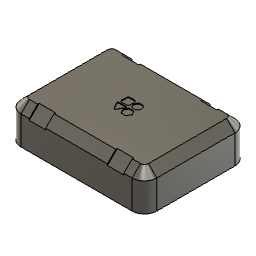
Bento Revised - Flat (Autodesk Fusion 360 design; units mm, degrees)
Autodesk Fusion 360 part; units mm, degrees
note: some values were not read from the file. Chosen so that the rebuilt part matches the saved one: which face or edge a step refers to.
sketch "Sketch1" plane through (0, 0, 0) normal (0, 1, 0) x (1, 0, 0)
  line L0 (82.5, 62.5) -> (-82.5, 62.5)
  line L1 (-82.5, 62.5) -> (-82.5, -62.5)
  line L2 (-82.5, -62.5) -> (82.5, -62.5)
  line L3 (82.5, -62.5) -> (82.5, 62.5)
  line L4 (82.5, 62.5) -> (-82.5, -62.5) construction
  line L5 (-82.5, 62.5) -> (82.5, -62.5) construction
  dimension "d1" = 165
  dimension "d2" = 125
  constraint horizontal L0
  constraint perpendicular L0 L1
  constraint parallel L0 L2
  constraint parallel L1 L3
  constraint coincident L4 origin
  constraint coincident L5 origin
  measures "d1" distance of L0.start L0.end
  measures "d2" distance of L0.start L2.end
extrude "Extrude1" add sketch "Sketch1" along normal blind 88 makes body 1
sketch "Sketch2" plane through (0, 0, 62.5) normal (0, 0, 1) x (1, 0, 0)
  line L0 (-82.5, 0) -> (82.5, 0)
  line L1 (82.5, 0) -> (82.5, 88)
  line L2 (82.5, 88) -> (-82.5, 88)
  line L3 (-82.5, 88) -> (-82.5, 0)
  line L4 (-28.95, 71.8572) -> (-48.25, 83)
  line L5 (-48.25, 83) -> (-67.55, 71.8572)
  line L6 (-67.55, 71.8572) -> (-67.55, 49.5714)
  line L7 (-67.55, 49.5714) -> (-48.25, 38.4286)
  line L8 (-48.25, 38.4286) -> (-28.95, 49.5714)
  line L9 (-28.95, 49.5714) -> (-28.95, 71.8572)
  circle A0 centre (-48.25, 60.7143) radius 22.2857 construction
  line L10 (-48.25, 60.7143) -> (-38.6, 44) construction
  line L11 (-48.25, 16.1428) -> (-28.95, 5)
  line L12 (-28.95, 5) -> (-9.65, 16.1428)
  line L13 (-9.65, 16.1428) -> (-9.65, 38.4286)
  line L14 (-9.65, 38.4286) -> (-28.95, 49.5714)
  line L15 (-28.95, 49.5714) -> (-48.25, 38.4286)
  line L16 (-48.25, 38.4286) -> (-48.25, 16.1428)
  line L17 (-28.95, 49.5714) -> (-9.65, 38.4286)
  line L18 (-9.65, 38.4286) -> (9.65, 49.5714)
  line L19 (9.65, 49.5714) -> (9.65, 71.8572)
  line L20 (9.65, 71.8572) -> (-9.65, 83)
  line L21 (-9.65, 83) -> (-28.95, 71.8572)
  line L22 (-28.95, 71.8572) -> (-28.95, 49.5714)
  line L23 (-9.65, 16.1428) -> (9.65, 5)
  line L24 (9.65, 5) -> (28.95, 16.1428)
  line L25 (28.95, 16.1428) -> (28.95, 38.4286)
  line L26 (28.95, 38.4286) -> (9.65, 49.5714)
  line L27 (9.65, 49.5714) -> (-9.65, 38.4286)
  line L28 (-9.65, 38.4286) -> (-9.65, 16.1428)
  line L29 (9.65, 49.5714) -> (28.95, 38.4286)
  line L30 (28.95, 38.4286) -> (48.25, 49.5714)
  line L31 (48.25, 49.5714) -> (48.25, 71.8572)
  line L32 (48.25, 71.8572) -> (28.95, 83)
  line L33 (28.95, 83) -> (9.65, 71.8572)
  line L34 (9.65, 71.8572) -> (9.65, 49.5714)
  line L35 (28.95, 16.1428) -> (48.25, 5)
  line L36 (48.25, 5) -> (67.55, 16.1428)
  line L37 (67.55, 16.1428) -> (67.55, 38.4286)
  line L38 (67.55, 38.4286) -> (48.25, 49.5714)
  line L39 (48.25, 49.5714) -> (28.95, 38.4286)
  line L40 (28.95, 38.4286) -> (28.95, 16.1428)
  line L41 (0, 77.4286) -> (0, 10.5714) construction
  line L42 (0, 0) -> (0, 88) construction
  line L43 (-82.5, 44) -> (82.5, 44) construction
  line L44 (-82.5, 44) -> (82.5, 44)
  line L45 (67.55, 38.4286) -> (67.55, 44)
  line L46 (57.9, 44) -> (57.9, 10.5714)
  point P0 (-48.25, 60.7143)
  dimension "d5" = 38.6
  dimension "d8" = 38.6
  dimension "d9" = 38.6
  dimension "d10" = 14.95
  dimension "d12" = 5
  dimension "d13" = 78
  constraint coincident P0 A0.centre
  constraint coincident L4.start A0
  constraint vertical L6
  constraint midpoint L8 L10.end
  constraint midpoint L20 L41.start
  constraint midpoint L23 L41.end
  constraint coincident L42.start origin
  constraint midpoint L2 L42.end
  constraint collinear L41 L42
  constraint midpoint L3 L43.start
  constraint midpoint L1 L43.end
  constraint midpoint L41 L43
  constraint coincident L43 L45.end
  constraint perpendicular L43 L45
  constraint midpoint L38 L46.start
  constraint coincident L36 L46.end
  constraint vertical L46
  measures "d5" distance of L6 L9
  measures "d10" distance of L1 L37
  measures "d12" distance of L2 L20.end
  measures "d13" vertical distance of L20.end L23.end
extrude "Extrude2" add sketch "Sketch2" against normal blind 105 from surface at -10 separate body contours L7 L8 L15 L44 | L4 L5 L6 L7 L8 L9 L15 L22 L44 | L8 L11 L12 L13 L14 L15 L16 L17 L28 L44 | L8 L14 L15 L17 L44 | L30 L38 L39 L44 | L25 L30 L35 L36 L39 L40 L44 L46 | L36 L37 L38 L46 | L9 L14 L17 L18 L19 L20 L21 L22 L27 L34 L44 | L14 L17 L18 L27 L44 | L19 L26 L29 L30 L31 L32 L33 L34 L39 L44 | L26 L29 L30 L39 L44 | L13 L18 L23 L24 L25 L26 L27 L28 L29 L40 L44 | L18 L26 L27 L29 L44 makes body 2
fillet "Fillet1" radius 5 18 edges at (28.95, 83, 0) (48.25, 71.8572, 0) (48.25, 49.5714, 0) (67.55, 38.4286, 0) (67.55, 16.1428, 0) (48.25, 5, 0) (-9.65, 83, 0) (9.65, 71.8572, 0) (-28.95, 71.8572, 0) (-48.25, 83, 0) (-67.55, 71.8572, 0) (-67.55, 49.5714, 0) (-48.25, 38.4286, 0) (-48.25, 16.1428, 0) (-28.95, 5, 0) (-9.65, 16.1428, 0) (9.65, 5, 0) (28.95, 16.1428, 0) on bodies 2
fillet "Fillet5" radius 15 4 edges at (82.5, 44, 62.5) (-82.5, 44, 62.5) (82.5, 44, -62.5) (-82.5, 44, -62.5) on bodies 1
chamfer "Chamfer4" distance 10.16 angle 45 16 edges at (78.1066, 88, 58.1066) (82.5, 88, 0) (78.1066, 88, -58.1066) (0, 88, -62.5) (-78.1066, 88, -58.1066) (-82.5, 88, 0) (-78.1066, 88, 58.1066) (0, 88, 62.5) (82.5, 0, 0) (78.1066, 0, -58.1066) (0, 0, -62.5) (-78.1066, 0, -58.1066) (-82.5, 0, 0) (-78.1066, 0, 58.1066) (0, 0, 62.5) (78.1066, 0, 58.1066) on bodies 1
combine "Combine1" operation cut target body 1 tool bodies 2
extrude "Extrude3" cut sketch "Sketch2" against normal blind 105 from surface at -10 contours L38 L44 L45 | L36 L37 L38 L46 bodies 1
extrude "Extrude4" cut sketch "Sketch2" against normal blind 125 contours L1 L2 L3 L4 L5 L6 L7 L20 L21 L31 L32 L33 L38 L44 | L4 L5 L6 L7 L8 L9 L15 L22 L44 | L8 L14 L15 L17 L44 | L30 L38 L39 L44 | L9 L14 L17 L18 L19 L20 L21 L22 L27 L34 L44 | L19 L26 L29 L30 L31 L32 L33 L34 L39 L44 | L18 L26 L27 L29 L44 bodies 1
fillet "Fillet3" radius 5 1 edges at (67.55, 16.1428, 0) on bodies 1
sketch "Sketch4" plane through (-82.5, 0, 0) normal (-1, 0, 0) x (0, 0, 1)
  line L0 (47.5, 44) -> (-47.5, 44)
  line L1 (0, 0) -> (-52.5, 0)
  line L2 (-62.5, 10) -> (-62.5, 44)
  line L3 (-62.5, 44) -> (62.5, 44)
  line L4 (62.5, 44) -> (62.5, 10)
  line L5 (52.5, 0) -> (0, 0)
  line L6 (54.3333, 42.5) -> (54.3333, 3.8333)
  line L7 (-54.8333, 42.5) -> (54.3333, 42.5)
  line L8 (-54.8333, 4.3333) -> (-54.8333, 42.5)
  line L9 (0, 0.0714) -> (-50.5714, 0.0714)
  line L10 (50.5714, 0.0714) -> (0, 0.0714)
  line L11 (54.3333, 42.5) -> (54.3333, 44)
  line L12 (-54.8333, 42.5) -> (-54.8333, 44)
  line L13 (-47.5, 44) -> (-47.5, 10.16)
  line L14 (-47.5, 10.16) -> (47.5, 10.16)
  line L15 (47.5, 10.16) -> (47.5, 44)
  line L16 (54.3333, 3.8333) -> (50.5714, 0.0714)
  line L17 (62.5, 10) -> (52.5, 0)
  line L18 (-54.8333, 4.3333) -> (-50.5714, 0.0714)
  line L19 (-62.5, 10) -> (-52.5, 0)
  line L20 (54.3333, 3.8333) -> (62.5, 12)
  line L21 (50.5714, 0.0714) -> (50.5, 0)
  line L22 (-50.5714, 0.0714) -> (-50.5, 0)
  line L23 (-54.8333, 4.3333) -> (-62.5, 12)
  point P0 (-62.5, 0)
  point P1 (62.5, 0)
  point P2 (0, 44)
  dimension "d38" = 44
  dimension "d39" = 44
  dimension "d40" = 125
  dimension "d70" = 10
  dimension "d71" = 2
  dimension "d72" = 45
  dimension "d73" = 45
  dimension "d74" = 10
  dimension "d75" = 2
  constraint coincident L1.start L5.end
  constraint horizontal L1
  constraint perpendicular L1 L2
  constraint perpendicular L2 L3
  constraint perpendicular L0 L4
  constraint perpendicular L4 L5
  constraint coincident P0 L2
  constraint coincident P0 L1
  constraint coincident P1 L5
  constraint coincident P1 L4
  constraint coincident L3 L11.end
  constraint perpendicular L3 L11
  constraint midpoint L3 P2
  constraint coincident L3 L12.end
  constraint perpendicular L3 L12
  constraint parallel L4 L6
  constraint parallel L3 L7
  constraint parallel L2 L8
  constraint parallel L1 L9
  constraint parallel L5 L10
  constraint coincident L4 L20.end
  constraint parallel L16 L20
  constraint coincident L5 L21.end
  constraint parallel L16 L21
  constraint coincident L1 L22.end
  constraint perpendicular L21 L22
  constraint coincident L2 L23.end
  constraint parallel L18 L23
  constraint parallel L17 L20
  constraint parallel L19 L23
  measures "d38" distance of L3.end P1
  measures "d39" distance of P0 L2.end
  measures "d40" distance of L2 L4
  measures "d70" vertical distance of L2.start L1.end
  measures "d71" distance of L2.start L23.end
  measures "d72" angle of L1 L19
  measures "d73" angle of L5 L17
  measures "d74" vertical distance of L5.start L4.end
  measures "d75" distance of L4.end L20.end
extrude "Extrude7" cut sketch "Sketch4" against normal blind 20 from surface at -25 contours L4 L5 L16 L17 L20 L21 | L1 L2 L18 L19 L22 L23 bodies 1
extrude "Extrude8" cut sketch "Sketch4" against normal blind 20 from surface at -120 contours L4 L5 L16 L17 L20 L21 | L1 L2 L18 L19 L22 L23 bodies 1
sketch "Sketch5" plane through (0, 44, 0) normal (0, 1, 0) x (-1, 0, 0)
  line L0 (-67.55, -52.5) -> (-67.55, 52.5)
  line L1 (-67.55, 52.5) -> (57.9, 52.5)
  line L2 (67.5, 62.5) -> (-67.5, 62.5)
  arc A0 (-67.5, 62.5) -> (-82.5, 47.5) centre (-67.5, 47.5) ccw
  line L3 (-82.5, 47.5) -> (-82.5, -47.5)
  arc A1 (-82.5, -47.5) -> (-67.5, -62.5) centre (-67.5, -47.5) ccw
  line L4 (-67.55, -25) -> (-82.5, -25)
  line L5 (-82.5, -25) -> (-82.5, 25)
  line L6 (-82.5, 25) -> (-67.55, 25)
  line L7 (-67.55, 25) -> (-67.55, -25)
  line L8 (0, -52.5) -> (0, 52.5)
  line L9 (82.5, 25) -> (67.55, 25)
  line L10 (67.55, 25) -> (67.55, -25)
  line L11 (67.55, -25) -> (82.5, -25)
  line L12 (82.5, -25) -> (82.5, 25)
  arc A2 (67.5, -62.5) -> (82.5, -47.5) centre (67.5, -47.5) ccw
  line L13 (82.5, -47.5) -> (82.5, 47.5)
  arc A3 (82.5, 47.5) -> (67.5, 62.5) centre (67.5, 47.5) ccw
  line L14 (57.9, 52.5) -> (57.9, -52.5)
  line L15 (0, -62.5) -> (0, -45)
  line L16 (0, 52.5) -> (0, 62.5)
  line L17 (67.55, 25) -> (67.55, 52.5)
  line L18 (67.55, 52.5) -> (0, 52.5)
  line L19 (0, -45) -> (-67.55, -45)
  line L20 (-67.55, -45) -> (-67.55, -25)
  line L21 (67.55, -25) -> (67.55, -45)
  line L22 (67.55, -45) -> (0, -45)
  line L23 (-67.55, 0) -> (-82.5, 0)
  line L24 (67.55, 0) -> (82.5, 0)
  line L25 (-67.5, -62.5) -> (67.5, -62.5)
  line L26 (57.9, -52.5) -> (-67.55, -52.5)
  line L27 (67.5, 62.5) -> (0, 62.5)
  dimension "d52" = 50
  constraint horizontal L4
  constraint vertical L5
  constraint horizontal L6
  constraint vertical L7
  constraint coincident L3 L5.end
  constraint coincident L0 L4.start
  constraint symmetric L4.start L8 L10.end
  constraint symmetric L4.end L8 L11.end
  constraint symmetric L5.end L8 L9.start
  constraint symmetric L6.end L8 L9.end
  constraint coincident L8 L15.end
  constraint coincident L1 L8.end
  constraint coincident L8 L16.start
  constraint midpoint L2 L16.end
  constraint perpendicular L1 L17
  constraint perpendicular L16 L18
  constraint perpendicular L0 L19
  constraint perpendicular L4 L20
  constraint midpoint L5 L23.end
  constraint midpoint L13 L24.end
  constraint coincident L10 L24.start
  constraint perpendicular L10 L24
  constraint coincident L0 L23.start
  constraint midpoint L3 L23.end
  constraint midpoint L7 L23.start
  constraint midpoint L15.start L25
  constraint horizontal L22
  constraint coincident L2.start A3.end
  measures "d52" distance of L4 L6
extrude "Extrude9" [suppressed]
extrude "Extrude11" [suppressed]
sketch "Sketch7" plane through (-67.55, 0, 0) normal (1, 0, 0) x (0, 0, -1)
  line L0 (-52.5, 44) -> (0, 44)
  line L1 (0, 44) -> (0, 49)
  line L2 (0, 49) -> (-52.5, 49)
  line L3 (-52.5, 49) -> (-52.5, 44)
  line L4 (-52.5, 49) -> (52.5, 49)
  line L5 (52.5, 49) -> (52.5, 39)
  line L6 (52.5, 39) -> (-52.5, 39)
  line L7 (-52.5, 39) -> (-52.5, 49)
  dimension "d82" = 105
  constraint horizontal L4
  constraint vertical L5
  constraint horizontal L6
  constraint vertical L7
  constraint coincident L2.end L3.start
  measures "d82" distance of L2.end L4.end
extrude "Extrude12" [suppressed]
chamfer "Chamfer1" [suppressed]
chamfer "Chamfer7" [suppressed]
chamfer "Chamfer8" [suppressed]
copy_body "CopyPasteBodies1" bodies 1 makes body 3
sketch "Sketch1 (2)" plane through (0, 0, 0) normal (0, 1, 0) x (1, 0, 0) in component "Logo v7 (1)"
  line L0 (5.725, 5.925) -> (-5.725, 5.925) construction
  line L1 (-5.725, 5.925) -> (-5.725, -5.925) construction
  line L2 (-5.725, -5.925) -> (5.725, -5.925) construction
  line L3 (5.725, -5.925) -> (5.725, 5.925) construction
  line L4 (5.725, 5.925) -> (-5.725, -5.925) construction
  line L5 (-5.725, 5.925) -> (5.725, -5.925) construction
  line L6 (-10.725, 10.925) -> (-0.725, 10.925)
  line L7 (-0.725, 10.925) -> (-0.725, 0.925)
  line L8 (-0.725, 0.925) -> (-10.725, 0.925)
  line L9 (-10.725, 0.925) -> (-10.725, 10.925)
  line L10 (-10.725, 10.925) -> (-0.725, 0.925) construction
  line L11 (-0.725, 10.925) -> (-10.725, 0.925) construction
  circle A0 centre (5.725, 5.925) radius 5
  circle A1 centre (-8.725, 8.925) radius 2
  circle A2 centre (-2.725, 8.925) radius 2
  circle A3 centre (-8.725, 2.925) radius 2
  circle A4 centre (-2.725, 2.925) radius 2
  line L12 (2.4132, -0.925) -> (-0.4735, -5.925)
  line L13 (-0.4735, -5.925) -> (2.4132, -10.925)
  line L14 (2.4132, -10.925) -> (8.1868, -10.925)
  line L15 (8.1868, -10.925) -> (11.0735, -5.925)
  line L16 (11.0735, -5.925) -> (8.1868, -0.925)
  line L17 (8.1868, -0.925) -> (2.4132, -0.925)
  line L18 (-5.725, -11.925) -> (0.6259, -0.925)
  line L19 (0.6259, -0.925) -> (-12.0759, -0.925)
  line L20 (-12.0759, -0.925) -> (-5.725, -11.925)
  circle A5 centre (-5.725, -4.5917) radius 7.3333 construction
  circle A6 centre (5.3, -5.925) radius 5.7735 construction
  circle A7 centre (-10.3438, -1.925) radius 1
  circle A8 centre (-1.1062, -1.925) radius 1
  circle A9 centre (-5.725, -9.925) radius 1
  circle A10 centre (0.5657, -5.925) radius 0.9
  circle A11 centre (2.9329, -1.825) radius 0.9
  circle A12 centre (7.6671, -1.825) radius 0.9
  circle A13 centre (10.0343, -5.925) radius 0.9
  circle A14 centre (7.6671, -10.025) radius 0.9
  circle A15 centre (2.9329, -10.025) radius 0.9
  line L21 (0.6259, -0.925) -> (2.4132, -0.925) construction
  point P0 (-5.725, 5.925)
  point P1 (5.3, -5.925)
  point P2 (-5.725, -4.5917)
  dimension "d1_2" = 11.45
  dimension "d2_2" = 11.85
  dimension "d3_2" = 10
  dimension "d4_2" = 10
  dimension "d5_2" = 10
  dimension "d10_2" = 4
  dimension "d11_1" = 4
  dimension "d12_2" = 4
  dimension "d13_2" = 4
  dimension "d14_2" = 0.425
  dimension "d15_2" = 10
  dimension "d18_1" = 1.8
  dimension "d19_2" = 1.8
  dimension "d20_2" = 1.8
  dimension "d21_2" = 1.8
  dimension "d22_2" = 1.8
  dimension "d23_2" = 1.8
  dimension "d24_2" = 2
  dimension "d25_2" = 2
  dimension "d26_1" = 2
  dimension "d29_2" = 9
  constraint perpendicular L0 L1
  constraint parallel L0 L2
  constraint parallel L1 L3
  constraint horizontal L0
  constraint coincident L4 origin
  constraint coincident L5 origin
  constraint perpendicular L6 L7
  constraint parallel L6 L8
  constraint parallel L7 L9
  constraint horizontal L6
  constraint coincident L10 P0
  constraint coincident L11 P0
  constraint coincident P0 L0.end
  constraint coincident L0.start L3.end
  constraint tangent L9 A1
  constraint tangent L6 A1
  constraint tangent L6 A2
  constraint tangent L7 A2
  constraint tangent L9 A3
  constraint tangent L8 A3
  constraint tangent L8 A4
  constraint tangent L7 A4
  constraint coincident P2 A5.centre
  constraint coincident L19.end A5
  constraint coincident P1 A6.centre
  constraint coincident L16.end A6
  constraint coincident L2 P1
  constraint horizontal L17
  constraint horizontal L19
  constraint coincident L1 P2
  constraint tangent L20 A7
  constraint tangent L19 A7
  constraint tangent L19 A8
  constraint tangent L18 A8
  constraint tangent L18 A9
  constraint tangent L20 A9
  constraint tangent L13 A10
  constraint tangent L12 A10
  constraint tangent L12 A11
  constraint tangent L17 A11
  constraint tangent L17 A12
  constraint tangent L16 A12
  constraint tangent L16 A13
  constraint tangent L15 A13
  constraint tangent L15 A14
  constraint tangent L14 A14
  constraint tangent L14 A15
  constraint tangent L13 A15
  constraint parallel L17 L21
  measures "d1_2" distance of L1 L3
  measures "d2_2" vertical distance of L0.start L2.end
  measures "d3_2" vertical distance of L6.start L8.end
  measures "d4_2" horizontal distance of L6.start L6.end
  measures "d5_2" diameter of A0
  measures "d10_2" diameter of A1
  measures "d11_1" diameter of A2
  measures "d12_2" diameter of A3
  measures "d13_2" diameter of A4
  measures "d14_2" horizontal distance of L2.end P1
  measures "d15_2" distance of L14 L17
  measures "d18_1" diameter of A10
  measures "d19_2" diameter of A11
  measures "d20_2" diameter of A12
  measures "d21_2" diameter of A13
  measures "d22_2" diameter of A14
  measures "d23_2" diameter of A15
  measures "d24_2" diameter of A8
  measures "d25_2" diameter of A7
  measures "d26_1" diameter of A9
  measures "d29_2" distance of L19 A9.centre
extrude "Extrude1'" add sketch "Sketch1 (2)" along normal blind 1 separate body contours L6 L7 L8 L9 A1 A2 A3 A4 | A1 | A2 | A3 | A4 | A0 | L12 L13 L14 L15 L16 L17 A10 A11 A12 A13 A14 A15 | A11 | A10 | A12 | A15 | A13 | A14 | L18 L19 L20 A7 A8 A9 | A9 | A8 | A7 makes body 4 at (4.7452, 0, -5.8516) makes body 5 at (-5.725, 0, 4.5917) makes body 6 at (-6.725, 0, -6.2583) makes body 7 at (6.089, 0, 7.5917) in component "Logo v7 (1)"
combine "Combine2" operation cut target body 3 tool bodies 6 4 7 5 body 6 seen with x (-1, 0, 0) y (0, -1, 0) z (0, 0, 1) at (0, 1, 0) body 4 seen with x (-1, 0, 0) y (0, -1, 0) z (0, 0, 1) at (0, 1, 0) body 7 seen with x (-1, 0, 0) y (0, -1, 0) z (0, 0, 1) at (0, 1, 0) body 5 seen with x (-1, 0, 0) y (0, -1, 0) z (0, 0, 1) at (0, 1, 0)
move_body "Move1" bodies 3 to x (-1, 0, 0) y (0, -1, 0) z (0, 0, 1) at (0, 88, 0)
extrude "Extrude13" add 1 faces at (66.1, 44, 15.8333) along direction (0, -1, 0) blind 1 on bodies 3 bodies 3
chamfer "Chamfer11" distance 1.73 angle 30 1 edges at (57.9, 43, 0) measured on face at (66.1, 43, 15.8333) on bodies 3
chamfer "Chamfer12" distance 1.5 angle 45 34 edges at (48.25, 60.7143, 52.5) (47.5801, 71.4704, 52.5) (38.6, 77.4286, 52.5) (28.95, 82.2265, 52.5) (19.3, 77.4286, 52.5) (9.65, 72.6307, 52.5) (0, 77.4286, 52.5) (-9.65, 82.2265, 52.5) (-19.3, 77.4286, 52.5) (-28.95, 72.6307, 52.5) (-38.6, 77.4286, 52.5) (-48.25, 82.2265, 52.5) (-57.9, 77.4286, 52.5) (-66.8801, 71.4704, 52.5) (-67.55, 55.9852, 52.5) (54.325, 46.064, 52.5) (48.9199, 49.9582, 52.5) (48.25, 60.7143, -52.5) (48.9199, 49.9582, -52.5) (54.325, 46.064, -52.5) (-67.55, 55.9852, -52.5) (-66.8801, 71.4704, -52.5) (-57.9, 77.4286, -52.5) (-48.25, 82.2265, -52.5) (-38.6, 77.4286, -52.5) (-28.95, 72.6307, -52.5) (-19.3, 77.4286, -52.5) (-9.65, 82.2265, -52.5) (0, 77.4286, -52.5) (9.65, 72.6307, -52.5) (19.3, 77.4286, -52.5) (28.95, 82.2265, -52.5) (38.6, 77.4286, -52.5) (47.5801, 71.4704, -52.5) measured on face at (48.25, 57.9623, 17.5) measured on face at (-3.1426, 54.9378, 52.5) measured on face at (40.9833, 76.0526, 17.5) measured on face at (-3.1426, 54.9378, 52.5) measured on face at (21.6833, 78.8046, -17.5) measured on face at (-3.1426, 54.9378, 52.5) measured on face at (2.3833, 76.0526, 17.5) measured on face at (-3.1426, 54.9378, 52.5) measured on face at (-16.9167, 78.8046, 17.5) measured on face at (-3.1426, 54.9378, 52.5) measured on face at (-36.2167, 76.0526, 17.5) measured on face at (-3.1426, 54.9378, 52.5) measured on face at (-60.2833, 76.0526, -17.5) measured on face at (-3.1426, 54.9378, 52.5) measured on face at (-67.55, 51.6568, -17.5) measured on face at (55.5167, 45.376, 17.5) measured on face at (-3.1426, 54.9378, 52.5) measured on face at (48.25, 57.9623, 17.5) measured on face at (-3.1426, 54.9378, -52.5) measured on face at (55.5167, 45.376, 17.5) measured on face at (-67.55, 51.6568, -17.5) measured on face at (-3.1426, 54.9378, -52.5) measured on face at (-60.2833, 76.0526, -17.5) measured on face at (-3.1426, 54.9378, -52.5) measured on face at (-36.2167, 76.0526, 17.5) measured on face at (-3.1426, 54.9378, -52.5) measured on face at (-16.9167, 78.8046, 17.5) measured on face at (-3.1426, 54.9378, -52.5) measured on face at (2.3833, 76.0526, 17.5) measured on face at (-3.1426, 54.9378, -52.5) measured on face at (21.6833, 78.8046, -17.5) measured on face at (-3.1426, 54.9378, -52.5) measured on face at (40.9833, 76.0526, 17.5) measured on face at (-3.1426, 54.9378, -52.5) on bodies 3
component "Logo v7 (1)" placed x (-1, 0, 0) y (0, -1, 0) z (0, 0, 1) at (0, 1, 0)
hidden bodies 1
equation "d1 = outerWidth"
equation "d2 = outerLength"
equation "d14 = -( outerLength - ( numBlinksInStack * blinkThickness ) ) / 2"
equation "d15 = -numBlinksInStack * blinkThickness"
equation "d19 = -( outerLength - ( numBlinksInStack * blinkThickness ) ) / 2"
equation "d20 = -( numBlinksInStack * blinkThickness )"
equation "d22 = -outerLength"
equation "d40 = outerLength"
equation "d43 = -bandOffset"
equation "d44 = -bandThickness"
equation "d46 = -outerWidth + bandOffset + bandThickness"
equation "d47 = -bandThickness"
equation "size = 10 mm"
equation "square_diameter = 0.4 * size"
equation "triangle_diameter = 0.2 * size"
equation "hexagon_diameter = 0.18 * size"
equation "d1_2 = size_1 * ( 1 + 0.145 )"
equation "d2_2 = size_1 * ( 1 + 0.185 )"
equation "d3_2 = size_1"
equation "d4_2 = size_1"
equation "d5_2 = size_1"
equation "size_1 = 10 mm"
equation "square_diameter_1 = 0.4 * size_1"
equation "triangle_diameter_1 = 0.2 * size_1"
equation "hexagon_diameter_1 = 0.18 * size_1"
equation "d10_2 = square_diameter_1"
equation "d11_1 = square_diameter_1"
equation "d12_2 = square_diameter_1"
equation "d13_2 = square_diameter_1"
equation "d14_2 = 0.0425 * size_1"
equation "d15_2 = size_1"
equation "d18_1 = hexagon_diameter_1"
equation "d19_2 = hexagon_diameter_1"
equation "d20_2 = hexagon_diameter_1"
equation "d21_2 = hexagon_diameter_1"
equation "d22_2 = hexagon_diameter_1"
equation "d23_2 = hexagon_diameter_1"
equation "d24_2 = triangle_diameter_1"
equation "d25_2 = triangle_diameter_1"
equation "d26_1 = triangle_diameter_1"
equation "d29_2 = size_1 - triangle_diameter_1 / 2"
equation "outerWidth = 165 mm"
equation "outerLength = 20 mm + numBlinksInStack * blinkThickness"
equation "blinkThickness = 15 mm"
equation "bandThickness = 20 mm"
equation "bandOffset = 25 mm"
equation "numBlinksInStack = 7"
equation "d82 = numBlinksInStack * blinkThickness"
named bodies: "bottom", "top"
